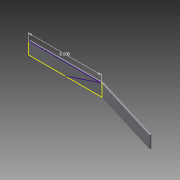
# Autodesk Inventor part: bent plough
Saved by Autodesk Inventor 2013 (Build 170138000, 138)
## iProperties
Created: 2013-02-07
Part Number: bent plough
Material: Generic
Document SubType Name: Sheet Metal
Designer: Arpan
Density: 1 g/cm^3
Sheet Metal Rule: Default
Author: Arpan
Autodesk Inventor part; units mm, degrees
ref_plane "YZ Plane" through (0, 0, 0) normal (1, 0, 0) x (0, 1, 0)
ref_plane "XZ Plane" through (0, 0, 0) normal (0, 1, 0) x (-1, 0, 0)
ref_plane "XY Plane" through (0, 0, 0) normal (0, 0, 1) x (1, 0, 0)
sketch "Sketch1" plane through (0, 0, 0) normal (0, 0, 1) x (1, 0, 0)
  line L0 (0, 0) -> (-154.1018, 0)
  line L1 (-154.1018, 0) -> (-154.1018, 25.4)
  line L2 (-154.1018, 25.4) -> (0, 25.4)
  line L3 (0, 25.4) -> (0, 0)
  dimension "d0" = 154.1018
  dimension "d1" = 25.4
  measures "d0" distance of L1.end L2.end
  measures "d1" distance of L2.end L0.start
extrude "Plate1" add sketch "Sketch1" along normal blind 3.175
sketch "Sketch2" plane through (0, 0, 3.175) normal (0, 0, 1) x (1, 0, 0)
  line L0 (-154.1018, 0) -> (-154.1018, 25.4) projected
  line L1 (0, 0) -> (-154.1018, 0) projected
  line L2 (0, 25.4) -> (0, 0) projected
  line L3 (-154.1018, 25.4) -> (0, 25.4) projected
  line L4 (-154.1018, 25.4) -> (-1.7018, 25.4)
  line L5 (-1.7018, 25.4) -> (-77.0509, 0)
  dimension "d3" = 152.4
  constraints: 4 end point, 1 midpoint, 1 point on line
  measures "d3" distance of L0.end L4.end
sketch "Sketch3" plane through (-0.9315, 25.4, 3.0353) normal (0.293373, 0, -0.9559981) x (0, 1, 0)
  line L0 (-25.4, 0) -> (0, 0)
  line L1 (0, 0) -> (0, 152.4)
  line L2 (0, 152.4) -> (-25.4, 152.4)
  line L3 (-25.4, 152.4) -> (-25.4, 0)
  constraints: 6 end point, 1 horizontal, 1 perpendicular, 1 vertical
edge flange "Flange1" height 152.4 angle 17.06 thickness 3.175 bend radius 1.27 thickness toward (0.293373, 0, -0.9559981) relief straight relief width 3.175 relief depth 1.5875 edges at (0, 12.7, 3.175) wall of the first edge with corners at (-0.9315, 0, 3.0353) (-0.9315, 25.4, 3.0353) (144.7626, 25.4, 47.7453) (144.7626, 0, 47.7453)
bend "Bend1"
corner "Corner1"
equation "\"d4\" = BendReliefWidth"
equation "\"d5\" = BendReliefDepth"
equation "\"d6\" = MinimumRemnant"
equation "\"d7\" = BendRadius"
equation "\"d11\" = CornerReliefSize"
equation "\"d12\" = GapSize"
equation "\"d13\" = JacobiRadiusSize"
equation "\"BendRadius\" = Thickness"
equation "\"BendReliefWidth\" = Thickness"
equation "\"BendReliefDepth\" = 0.5 * Thickness"
equation "\"CornerReliefSize\" = 4 * Thickness"
equation "\"MinimumRemnant\" = 2 * Thickness"
equation "\"TransitionRadius\" = BendRadius"
equation "\"JacobiRadiusSize\" = Thickness"
equation "\"GapSize\" = Thickness"
equation "\"d2\" = BendRadius"
equation "\"Thickness\" = 3.175"
body "Solid1"
